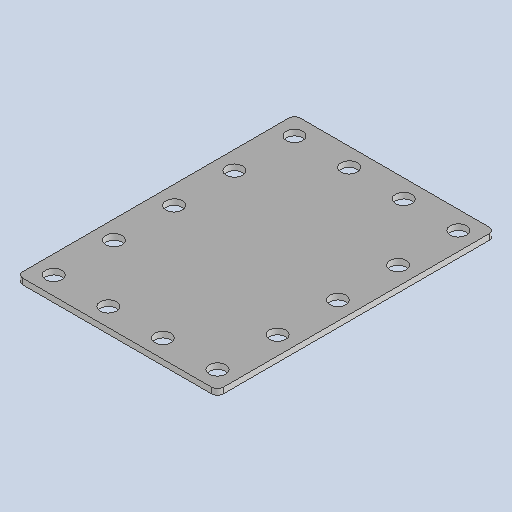
# Autodesk Inventor part: PRS 9607 charging flange rect_D1200 940
Saved by Autodesk Inventor 2026.2 (Build 302298000, 298)
## iProperties
Created: 2025-02-13
Part Number: PRS 9607 charging flange rect_D1200 940
Material: Steel
Document SubType Name: Sheet Metal
Designer: admin
Mass: 2466.79 g
Surface Area: 934.137 cm^2
Volume: 314.241 cm^3
Density: 7.85 g/cm^3
Flat Pattern Width: 28.8 cm
Flat Pattern Length: 20.8 cm
Flat Pattern Area: 599.04 cm^2
Sheet Metal Rule: AISI304 4mm Die 32
Sheet Metal Width: 288,000 mm
Sheet Metal Length: 208,000 mm
Sheet Metal Area: 59904,000 mm^2
Appearance: Default
Author: pokla
Autodesk Inventor part; units mm, degrees
ref_plane "YZ Plane" through (0, 0, 0) normal (1, 0, 0) x (0, 1, 0)
ref_plane "XZ Plane" through (0, 0, 0) normal (0, 1, 0) x (-1, 0, 0)
ref_plane "XY Plane" through (0, 0, 0) normal (0, 0, 1) x (1, 0, 0)
sketch "Sketch2" plane through (0, 0, 0) normal (0, 0, 1) x (1, 0, 0)
  line L0 (-54, -94) -> (54, -94)
  line L1 (54, -94) -> (54, 94)
  line L2 (54, 94) -> (-54, 94)
  line L3 (-54, 94) -> (-54, -94)
  line L4 (-54, -94) -> (54, 94) construction
  line L5 (54, -94) -> (-54, 94) construction
  line L6 (-104, -144) -> (104, -144)
  line L7 (104, -144) -> (104, 144)
  line L8 (104, 144) -> (-104, 144)
  line L9 (-104, 144) -> (-104, -144)
  point P0 (0, 0)
  dimension "d31" = 50
  dimension "d60" = 188
  dimension "d61" = 108
  measures "d31" distance between parallel lines of L3 L9
  measures "d60" distance of L2.end L0.start
  measures "d61" distance of L0.start L0.end
extrude "Plate2" add sketch "Sketch2" along normal blind 6 contours L3 L2 L1 L0 | L9 L8 L7 L6
sketch "Sketch5" plane through (0, 0, 6) normal (0, 0, 1) x (1, 0, 0)
  line L0 (104, -144) -> (-104, -144) construction
  line L1 (104, 144) -> (104, -144) construction
  line L2 (-104, 144) -> (104, 144) construction
  line L3 (-104, -144) -> (-104, 144) construction
  line L4 (-85, 125) -> (85, 125) construction
  line L5 (85, 125) -> (85, -125) construction
  line L6 (85, -125) -> (-85, -125) construction
  line L7 (-85, -125) -> (-85, 125) construction
  line L8 (-28.3333, -125) -> (28.3333, -125)
  line L9 (28.3333, -125) -> (28.3333, 125) construction
  line L10 (28.3333, 125) -> (-28.3333, 125)
  line L11 (-28.3333, 125) -> (-28.3333, -125) construction
  line L12 (-28.3333, 0) -> (28.3333, 0) construction
  point P0 (0, 0)
  point P1 (0, -125)
  point P2 (-85, -62.5)
  point P3 (-85, 0)
  point P4 (-85, 62.5)
  point P5 (85, 62.5)
  point P6 (85, 0)
  point P7 (85, -62.5)
  point P8 (0, 0)
  dimension "d34" = 19
  dimension "d47" = 62.5
  dimension "d48" = 62.5
  dimension "d49" = 56.6667
  dimension "d50" = 56.6667
  constraints: 18 end point, 8 point on line, 6 midpoint, 5 coincident, 2 parallel, 2 symmetric about line, 1 horizontal, 1 horizontal alignment, 1 perpendicular, 3 other
  measures "d34" distance between parallel lines of L0 L6
  measures "d47" distance of point (-85, -62.5) point (-85, -125)
  measures "d48" distance of point (-85, 0) point (-85, -62.5)
  measures "d49" distance of L8.start point (-85, -125)
  measures "d50" distance of L8.end L8.start
fillet "Corner Round1" radius 6 4 edges at (-104, -144, 3) (-104, 144, 3) (104, 144, 3) (104, -144, 3)
hole "Hole1" at (-85, -125, 6) at (-85, -62.5, 6) at (-85, 0, 6) at (-85, 62.5, 6) at (-85, 125, 6) at (85, 125, 6) at (85, 62.5, 6) at (85, 0, 6) at (85, -62.5, 6) at (85, -125, 6) at (-28.3333, -125, 6) at (28.3333, 125, 6) at (28.3333, -125, 6) at (-28.3333, 125, 6) direction (0, 0, -1) diameter 17 end through all
equation "\"d47\" = d48"
equation "\"d49\" = d50"
equation "\"d60\" = ChargingHatch_width - 2 * Thickness"
equation "\"d61\" = ChargingHatch_hight - 2 * Thickness"
equation "\"d56\" = Thickness"
equation "\"d14\" = Thickness"
equation "\"BendReliefWidth\" = Thickness"
equation "\"BendReliefDepth\" = 0.5 * Thickness"
equation "\"CornerReliefSize\" = 4 * Thickness"
equation "\"MinimumRemnant\" = 2 * Thickness"
equation "\"TransitionRadius\" = BendRadius"
equation "\"JacobiRadiusSize\" = BendRadius"
equation "\"GapSize\" = Thickness"
equation "\"ChargingHatch_width\" = 200"
equation "\"Thickness\" = 6"
equation "\"ChargingHatch_hight\" = 120"
equation "\"BendRadius\" = 6"
body "Solid3"
